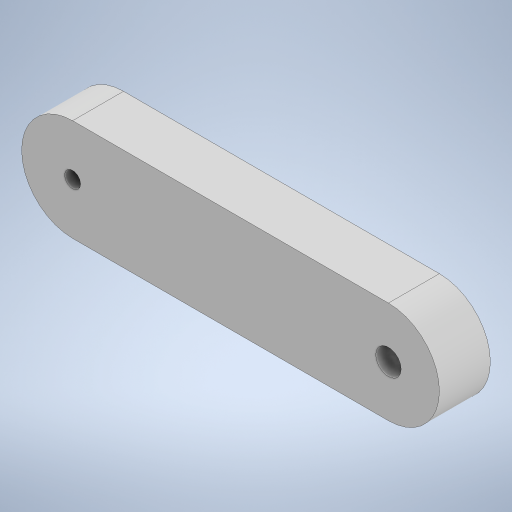
# Autodesk Inventor part: bunny neck
Saved by Autodesk Inventor 2024.2 (Build 282272000, 272)
## iProperties
Created: 2025-12-17
Part Number: bunny neck
Material: Generic
Document SubType Name: Modeling
Designer: David Toler II
Density: 1 g/cm^3
Appearance: Default
Author: David Toler II
Autodesk Inventor part; units mm, degrees
ref_plane "YZ Plane" through (0, 0, 0) normal (1, 0, 0) x (0, 1, 0)
ref_plane "XZ Plane" through (0, 0, 0) normal (0, 1, 0) x (-1, 0, 0)
ref_plane "XY Plane" through (0, 0, 0) normal (0, 0, 1) x (1, 0, 0)
sketch "Sketch1" plane through (0, 0, 0) normal (0, 0, 1) x (1, 0, 0)
  line L0 (19.685, 0) -> (-19.685, 0) construction
  line L1 (19.685, 6.35) -> (-19.685, 6.35)
  line L2 (-19.685, -6.35) -> (19.685, -6.35)
  arc A0 (19.685, -6.35) -> (19.685, 6.35) centre (19.685, 0) ccw
  arc A1 (-19.685, 6.35) -> (-19.685, -6.35) centre (-19.685, 0) ccw
  circle A2 centre (-19.685, 0) radius 3.175
  circle A3 centre (19.685, 0) radius 1.5875
  point P0 (0, 0)
  dimension "d0" = 6.35
  dimension "d1" = 39.37
  dimension "d2" = 6.35
  dimension "d3" = 3.175
  constraints: 8 end point, 4 centre point, 4 point on circle, 4 tangent, 2 coincident, 1 horizontal, 1 midpoint, 1 parallel
  measures "d0" radius of A1
  measures "d1" distance of L0.start L0.end
  measures "d2" diameter of A2
  measures "d3" diameter of A3
extrude "Extrusion1" add sketch "Sketch1" along normal blind 3.175
sketch "Sketch2" plane through (0, 0, 3.175) normal (0, 0, 1) x (1, 0, 0)
  arc A0 (-19.685, 6.35) -> (-19.685, -6.35) centre (-19.685, 0) ccw projected
  line L0 (-19.685, -6.35) -> (19.685, -6.35) projected
  arc A1 (19.685, -6.35) -> (19.685, 6.35) centre (19.685, 0) ccw projected
  line L1 (19.685, 6.35) -> (-19.685, 6.35) projected
  circle A2 centre (19.685, 0) radius 1.5875 projected
  circle A3 centre (-19.685, 0) radius 3.175 projected
  circle A4 centre (-19.685, 0) radius 1
  point P0 (0, 0)
  dimension "d6" = 2
  constraints: 1 centre point, 1 coincident
  measures "d6" diameter of A4
extrude "Extrusion2" add sketch "Sketch2" along normal blind 3.175 contours L1 A1 L0 A0 | A3
body "Solid1"
